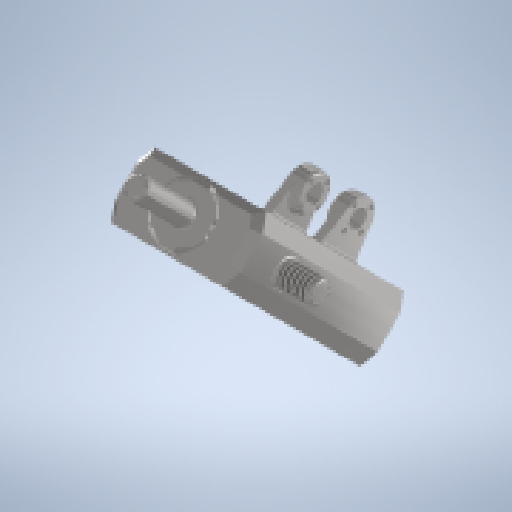
# Autodesk Inventor part: robot_tool_arm
Saved by Autodesk Inventor 2023 (Build 270158000, 158)
## iProperties
Created: 2023-11-20
Part Number: robot_tool_arm
Material: Steel, Mild
Document SubType Name: Modeling
Designer: Beatrice
Density: 7.85 g/cm^3
Appearance: Semi-Polished
Author: Beatrice
Autodesk Inventor part; units mm, degrees
sketch "Sketch1" plane through (0, 0, 0) normal (1, 0, 0) x (0, 1, 0)
  line L0 (0.000631, 41.00085) -> (0, 41.00085) construction
  ellipse E0 centre (0, 6.241435) end of major axis (6.25, 6.241435) minor radius 6.241435 (-6.242267, 6.551818) -> (6.239344, 6.605742) ccw construction
  ellipse E1 centre (0, 6.241435) end of major axis (-5, 6.241435) minor radius 5 construction
  line L1 (2.467238, 42.251676) -> (-2.456164, 42.251676) construction
  ellipse E2 centre (0, 47.251435) end of major axis (4.2185, 47.251435) minor radius 4.212719 (4.2185, 47.251435) -> (-4.2185, 47.251435) ccw construction
  ellipse E3 centre (0, 47.251435) end of major axis (-3, 47.251435) minor radius 3 (0.022533, 44.251519) -> (-0.022533, 44.251519) ccw construction
  line L2 (-4.20992, 47.251435) -> (-6.25, 6.241435) construction
  line L3 (4.221488, 47.251435) -> (6.244832, 6.495206) construction
  line L4 (-6.001619, 11.234435) -> (6.009553, 11.234435) construction
  line L5 (-2.456164, 42.251676) -> (-3.942535, 12.372435) construction
  line L6 (-3.942535, 12.372435) -> (3.950593, 12.372435) construction
  line L7 (-2.456674, 42.241435) -> (2.467746, 42.241435) construction
  line L8 (0.000627, 41.000095) -> (0, 41.000095) construction
  line L9 (2.467238, 42.251676) -> (3.950593, 12.372435) construction
  line L10 (-4.2185, 47.251435) -> (-4.20992, 47.251435) construction
  line L11 (0, 48.389405) -> (0, 48.389405) construction
  line L12 (3, 47.251435) -> (4.2185, 47.251435) construction
  line L13 (-19.109149, 33.389405) -> (19.109149, 33.389405) construction
  line L14 (-15.949888, 49.339293) -> (15.949888, 17.439516) construction
  line L15 (-15.99534, 17.394065) -> (15.99534, 49.384745) construction
  circle A0 centre (0, 47.251435) radius 3 construction
  circle A1 centre (0, 47.251435) radius 4.2185 construction
  line L16 (18.23022, 47.251435) -> (-40.280659, 47.251435) construction
  line L17 (-28.915137, 45.562681) -> (-28.915137, 48.940188) construction
  line L18 (0, 51.469935) -> (0, 43.032935) construction
  line L19 (0, 43.032935) -> (-28.915137, 45.562681) construction
  line L20 (0, 51.469935) -> (-28.915137, 48.940188) construction
  line L21 (-1.091828, 51.326193) -> (-28.366959, 41.398857) construction
  line L22 (-27.492796, 38.136436) -> (-28.366959, 41.398857) construction
  line L23 (1.091828, 43.176676) -> (-27.492796, 38.136436) construction
  line L24 (17.60904, 51.969763) -> (-38.908129, 36.826033) construction
  line L25 (-1.091828, 51.326193) -> (1.091828, 43.176676) construction
  line L26 (-11.845739, 45.235144) -> (-12.729622, 44.35126) construction
  line L27 (-12.729622, 44.35126) -> (-10.961855, 42.583493) construction
  line L28 (-10.961855, 42.583493) -> (-10.077972, 43.467377) construction
  line L29 (-11.845739, 45.235144) -> (-10.961855, 46.119027) construction
  line L30 (-10.961855, 46.119027) -> (-9.194088, 44.35126) construction
  line L31 (-9.194088, 44.35126) -> (-10.077972, 43.467377) construction
  line L32 (-34.002813, 47.251435) -> (-25.278291, 38.526913) construction
  line L33 (-21.561378, 39.182305) -> (-22.707266, 43.458817) construction
  line L34 (-28.188696, 40.733572) -> (-22.393141, 42.286487) construction
  line L35 (-27.671058, 38.801721) -> (-21.875503, 40.354635) construction
  line L36 (-13.402845, 41.866428) -> (-9.161157, 46.108116) construction
  circle A2 centre (-9.161157, 46.108116) radius 0.5 construction
  circle A3 centre (-9.161157, 46.108116) radius 0.9 construction
  line L37 (-10.961855, 46.119027) -> (-9.606243, 46.890355) construction
  line L38 (-9.194088, 44.35126) -> (-8.396947, 45.63274) construction
  line L39 (-12.729622, 44.35126) -> (-13.50095, 42.995648) construction
  circle A4 centre (-12.718711, 42.550562) radius 0.9 construction
  circle A5 centre (-12.718711, 42.550562) radius 0.5 construction
  line L40 (-10.961855, 42.583493) -> (-12.243335, 41.786351) construction
  line L41 (-28.188696, 40.733572) -> (-33.018325, 39.439477) construction
  line L42 (-33.018325, 39.439477) -> (-32.500687, 37.507625) construction
  line L43 (-32.500687, 37.507625) -> (-27.671058, 38.801721) construction
  circle A6 centre (-32.759506, 38.473551) radius 1.01 construction
  circle A7 centre (-32.759506, 38.473551) radius 0.639812 construction
  line L44 (-42.889211, 48.603256) -> (-22.629802, 28.343847) construction
  circle A8 centre (-32.759506, 38.473551) radius 0.639812
  circle A9 centre (-32.759506, 38.473551) radius 1.25
  line L45 (-33.64339, 39.357435) -> (-31.875623, 37.589668)
  line L46 (-31.875623, 37.589668) -> (-33.289836, 36.175454)
  line L47 (-33.289836, 36.175454) -> (-35.057603, 37.943221)
  line L48 (-35.057603, 37.943221) -> (-33.64339, 39.357435)
  circle A10 centre (-33.018325, 39.439477) radius 0.2
  circle A11 centre (-33.725432, 38.214732) radius 0.2
  circle A12 centre (-32.500687, 37.507625) radius 0.2
  circle A13 centre (-31.793581, 38.73237) radius 0.2
  line L49 (-31, 33.885618) -> (-41.606602, 44.49222)
  line L50 (-44.736864, 41.361957) -> (-34.130262, 30.755356)
  line L51 (-34.130262, 30.755356) -> (-31, 33.885618)
  line L52 (-33.64339, 39.357435) -> (-35.436541, 38.322159)
  line L53 (-33.64339, 39.357435) -> (-31.572837, 39.357435) construction
  line L54 (-31.875623, 37.589668) -> (-32.910899, 35.796517)
  line L55 (-35.436541, 38.322159) -> (-32.910899, 35.796517)
  line L56 (-32.910899, 35.796517) -> (-33.866631, 34.840785)
  line L57 (-33.866631, 34.840785) -> (-36.392273, 37.366427)
  line L58 (-36.392273, 37.366427) -> (-35.436541, 38.322159)
  line L59 (-41.606602, 44.49222) -> (-44.736864, 41.361957)
  line L60 (-43.171733, 42.927088) -> (-32.565131, 32.320487) construction
  line L61 (-43.171733, 42.927088) -> (-45.236644, 44.992) construction
  point P0 (0, 0)
  point P1 (28.751869, 36.37116)
  point P2 (0, 0)
  point P3 (0, 12.372435)
  point P4 (-6.009, 41)
  point P5 (0, 33.389405)
  point P6 (0, 47.251435)
  point P7 (0, 47.251435)
  dimension "d10" = 3
  dimension "d11" = 5
  dimension "d12" = 6.24143
  dimension "d2" = 41.01
  dimension "d3" = 6.24143
  dimension "d4" = 4.993
  dimension "d5" = 5.69
  dimension "d6" = 29.869
  dimension "d7" = 1.138
  dimension "d8" = 2
  dimension "d9" = 90
  dimension "d13" = 15
  dimension "d14" = 2.5
  dimension "d15" = 1.25
  dimension "d16" = 60
  dimension "d17" = 2
  dimension "d18" = 1
  dimension "d19" = 6
  dimension "d20" = 1
  dimension "d21" = 1.8
  dimension "d22" = 5
  dimension "d23" = 2
  dimension "d24" = 2.02
  dimension "d25" = 2.5
  dimension "d26" = 0.4
  dimension "d29" = 360
  dimension "d31" = 150
  dimension "d32" = 15
  dimension "d35" = 15
  constraints: 124 end point, 23 point on line, 14 parallel, 13 centre point, 12 coincident, 8 midpoint, 8 perpendicular, 7 symmetric about line, 6 point on circle, 3 collinear, 3 horizontal, 2 horizontal alignment, 2 tangent, 1 concentric, 1 equal length, 1 vertical alignment, 49 other
  measures "d2" distance of point (0, 47.251) point (0, 6.241)
  measures "d3" distance of point (0, 0) point (0, 6.241)
  measures "d4" distance from line of point (0, 6.241) L4
  measures "d5" angle of L2 L3
  measures "d6" distance between parallel lines of L6 L7
  measures "d7" distance between parallel lines of L4 L6
  measures "d8" distance between parallel lines of L2 L5
  measures "d9" angle of L14 L15
  measures "d14" distance between parallel lines of L26 L28
  measures "d15" distance between parallel lines of L14 L27
  measures "d16" angle of L32 L24
  measures "d17" distance between parallel lines of L35 L34
  measures "d18" distance between parallel lines of L34 L24
  measures "d19" distance between parallel lines of L33 L22
  measures "d20" diameter of A2
  measures "d21" diameter of A3
  measures "d22" distance between parallel lines of L42 L22
  measures "d23" distance of L45.end L46.end
  measures "d24" diameter of A6
  measures "d25" diameter of A9
  measures "d26" diameter of A10
  measures "d31" angle of L52 L53
  measures "d32" angle of L54 L46
  measures "d35" distance between parallel lines of L51 L59
extrude "Extrusion1" add sketch "Sketch1" against normal blind 3 contours L47 L49 L56 L57 L58 | L58 L57 L56 L49 L51 L50 L59
extrude "Extrusion2" add sketch "Sketch1" against normal blind 0.6 contours A8 L45 A9 | A8 L45 A9 | A9 L46 L47 L48 | L48 L49 L52 | L54 L49 L46
extrude "Extrusion3" add sketch "Sketch1" along normal blind 0.5 contours A8 L45 A9 | A8 L45 A9
extrude "Extrusion4" add sketch "Sketch1" along normal blind 1.5 contours L47 L49 L56 L57 L58 | L58 L57 L56 L49 L51 L50 L59
ref_plane "Work Plane1" through (1.5, 0, 0) normal (1, 0, 0) x (0, 0, -1)
mirror "Mirror1" about plane through (1.5, 0, 0) normal (1, 0, 0) of "Extrusion1", "Extrusion2", "Extrusion3", "Extrusion4"
chamfer "Chamfer1" distance 0.5 angle 65 3 edges at (6, -32.1449, 35.0305) (6, -38.3321, 41.2177) (6, -34.1737, 37.0593) measured on face at (5.5, -34.1737, 37.0593) measured on face at (5.5, -32.1449, 35.0305) measured on face at (5.5, -38.3321, 41.2177)
chamfer "Chamfer2" distance 0.5 angle 65 1 edges at (-3, -36.3033, 39.1889) measured on face at (-2.5, -36.3033, 39.1889)
chamfer "Chamfer3" distance 0.5 angle 65 1 edges at (6, -39.4336, 36.0587) measured on face at (5.5, -39.4336, 36.0587)
chamfer "Chamfer4" distance 0.5 angle 65 1 edges at (-3, -39.4336, 36.0587) measured on face at (-2.5, -39.4336, 36.0587)
chamfer "Chamfer5" distance 0.5 angle 45 28 edges at (-1.25, -41.6066, 44.4922) (0.75, -41.6066, 44.4922) (2.25, -41.6066, 44.4922) (4.25, -41.6066, 44.4922) (-1.25, -44.7369, 41.362) (0.75, -44.7369, 41.362) (2.25, -44.7369, 41.362) (4.25, -44.7369, 41.362) (-2.75, -44.3578, 41.7411) (-3, -43.1717, 42.9271) (-2.75, -41.9857, 44.1131) (5.75, -44.3578, 41.7411) (6, -43.1717, 42.9271) (5.75, -41.9857, 44.1131) (6, -32.5651, 32.3205) (5.75, -31.3791, 33.5065) (-1.25, -31, 33.8856) (0.75, -31, 33.8856) (2.25, -31, 33.8856) (4.25, -31, 33.8856) (-2.75, -31.3791, 33.5065) (-3, -32.5651, 32.3205) (-2.75, -33.7512, 31.1345) (-1.25, -34.1303, 30.7554) (0.75, -34.1303, 30.7554) (2.25, -34.1303, 30.7554) (4.25, -34.1303, 30.7554) (5.75, -33.7512, 31.1345)
sketch "Sketch2" plane through (-2.181465, -41.960155, 44.138666) normal (0, -0.7071068, 0.7071068) x (1, 0, 0)
  line L0 (0, 0) -> (7.36293, 0)
  line L1 (-0.318535, -0.683101) -> (0, 0)
  line L2 (-0.318535, -2.743759) -> (-0.318535, -0.683101)
  line L3 (0, -3.426859) -> (-0.318535, -2.743759)
  line L4 (7.36293, -3.426859) -> (0, -3.426859)
  line L5 (7.681465, -2.743759) -> (7.36293, -3.426859)
  line L6 (7.681465, -0.683101) -> (7.681465, -2.743759)
  line L7 (7.36293, 0) -> (7.681465, -0.683101)
  line L8 (-0.318535, -0.683101) -> (-0.318535, -2.743759)
  line L9 (-0.318535, -1.71343) -> (7.681465, -1.71343) construction
  line L10 (7.681465, -2.743759) -> (7.681465, -0.683101)
  line L11 (7.36293, 0) -> (0, 0)
  line L12 (3.681465, 0) -> (3.681465, -3.426859) construction
  line L13 (0, -3.426859) -> (7.36293, -3.426859)
  circle A0 centre (3.681465, -1.71343) radius 0.75
  circle A1 centre (3.681465, -1.71343) radius 2
  point P0 (2.181465, -1.54044)
  dimension "d60" = 1.5
  dimension "d61" = 4
  constraints: 5 midpoint, 4 end point, 2 centre point, 1 coincident
  measures "d60" diameter of A0
  measures "d61" diameter of A1
extrude "Extrusion5" add sketch "Sketch2" along normal blind 5 and the other way blind 1 contours A0
ref_plane "Work Plane2" through (-2.181465, -41.606602, 43.785113) normal (0, -0.7071068, 0.7071068) x (1, 0, 0)
sketch "Sketch3" plane through (-2.181465, -41.606602, 43.785113) normal (0, -0.7071068, 0.7071068) x (1, 0, 0)
  circle A0 centre (3.681465, -1.71343) radius 2
  circle A1 centre (3.681465, -1.71343) radius 0.75
  circle A2 centre (3.681465, -1.71343) radius 0.75
  circle A3 centre (3.681465, -1.71343) radius 1.826556
  line L0 (3.681465, 0.376831) -> (3.681465, -1.71343) construction
  line L1 (-0.677885, 0.238075) -> (7.322115, 0.238075) construction
  line L2 (7.36293, 0) -> (0, 0)
  line L3 (3.048642, 0) -> (3.24371, 0.238075)
  line L4 (3.24371, 0.238075) -> (4.11922, 0.238075)
  line L5 (4.11922, 0.238075) -> (4.314288, 0)
  line L6 (-0.188263, -4.512985) -> (3.811737, 2.415218) construction
  line L7 (2.210289, -0.358571) -> (2.514003, -0.308674)
  line L8 (1.88118, -1.404755) -> (1.772535, -1.116784)
  line L9 (1.772535, -1.116784) -> (2.210289, -0.358571)
  line L10 (4.171087, -6.46449) -> (0.171087, 0.463713) construction
  line L11 (1.772535, -2.310075) -> (1.88118, -2.022104)
  line L12 (2.514003, -3.118185) -> (2.210289, -3.068289)
  line L13 (2.210289, -3.068289) -> (1.772535, -2.310075)
  line L14 (8.040815, -3.664934) -> (0.040815, -3.664934) construction
  line L15 (3.24371, -3.664934) -> (3.048642, -3.426859)
  line L16 (4.314288, -3.426859) -> (4.11922, -3.664934)
  line L17 (4.11922, -3.664934) -> (3.24371, -3.664934)
  line L18 (7.551193, 1.086126) -> (3.551193, -5.842077) construction
  line L19 (5.15264, -3.068289) -> (4.848927, -3.118185)
  line L20 (5.48175, -2.022104) -> (5.590395, -2.310075)
  line L21 (5.590395, -2.310075) -> (5.15264, -3.068289)
  line L22 (3.191842, 3.037631) -> (7.191842, -3.890572) construction
  line L23 (5.590395, -1.116784) -> (5.48175, -1.404755)
  line L24 (4.848927, -0.308674) -> (5.15264, -0.358571)
  line L25 (5.15264, -0.358571) -> (5.590395, -1.116784)
  circle A4 centre (3.681465, -1.71343) radius 2.083382
  point P0 (2.181465, -1.54044)
  point P1 (4.848927, -0.308674)
  point P2 (5.48175, -1.404755)
  point P3 (5.48175, -2.022104)
  point P4 (4.848927, -3.118185)
  point P5 (2.514003, -3.118185)
  point P6 (1.88118, -2.022104)
  point P7 (2.514003, -0.308674)
  dimension "d69" = 360
  constraints: 50 end point, 13 point on line, 4 point on circle, 2 centre point, 2 coincident, 1 vertical, 61 other
extrude "Extrusion6" cut sketch "Sketch3" along normal blind 5 and the other way blind 5 contours A0 L20 A3 L23 | A0 L2 A4 | L25 A0 | A0 L21 | L24 A3 L2 A0 | A0 L16 A3 L19 | L2 L5 A0 | A0 L2 A4 | A0 L17 | L4 A0 | A0 L12 A3 L15 | L3 L2 A0 | A3 L7 A0 L2 | A0 L13 | A0 L8 A3 L11 | L9 A0
chamfer "Chamfer6" distance 0.2 angle 45 1 edges at (0.75, -46.7073, 46.4626)
fillet "Fillet1" radius 0.2 1 edges at (0.75, -43.1717, 42.9271)
fillet "Fillet2" radius 0.2 12 edges at (-0.6, -34.1737, 37.0593) (-0.3, -35.4365, 38.3222) (3, -34.1737, 37.0593) (3.3, -35.4365, 38.3222) (3.3, -32.9109, 35.7965) (-0.3, -32.9109, 35.7965) (3.6, -34.1737, 37.0593) (0, -34.1737, 37.0593) (3, -33.6434, 37.5897) (2.5, -34.0095, 38.4736) (0, -33.6434, 37.5897) (0.5, -34.0095, 38.4736)
sketch "Sketch4" plane through (6, -42.011246, 43.380468) normal (1, 0, 0) x (0, -0.7071068, -0.7071068)
  line L0 (0, 14) -> (2.282352, 14)
  line L1 (0, 0) -> (0, 14)
  line L2 (2.282352, 0) -> (0, 0)
  line L3 (2.282352, 14) -> (2.282352, 0)
  line L4 (0, 0) -> (2.282352, 0)
  line L5 (1.141176, 0) -> (1.141176, 14) construction
  line L6 (0, 3.5) -> (2.282352, 3.5) construction
  circle A0 centre (1.141176, 3.5) radius 0.8
  line L7 (0.110847, -0.5) -> (2.171505, -0.5)
  point P0 (0.968186, 60.38106)
  dimension "d80" = 3.5
  dimension "d81" = 1.6
  constraints: 4 end point, 3 midpoint, 2 point on line, 1 centre point, 1 horizontal
  measures "d80" distance between parallel lines of L6 L2
  measures "d81" diameter of A0
extrude "Extrusion7" add sketch "Sketch4" along normal blind 2.5 contours A0
fillet "Fillet3" radius 0.2 2 edges at (6, -39.7776, 40.6643) (8.5, -39.7776, 40.6643)
thread "Thread1" size "M1.6x0.35" class "6g" standard "ANSI Metric M Profile" full length
ref_plane "Work Plane3" through (1.5, -42.011246, 43.380468) normal (1, 0, 0) x (0, -0.7071068, -0.7071068)
body "Solid1"
